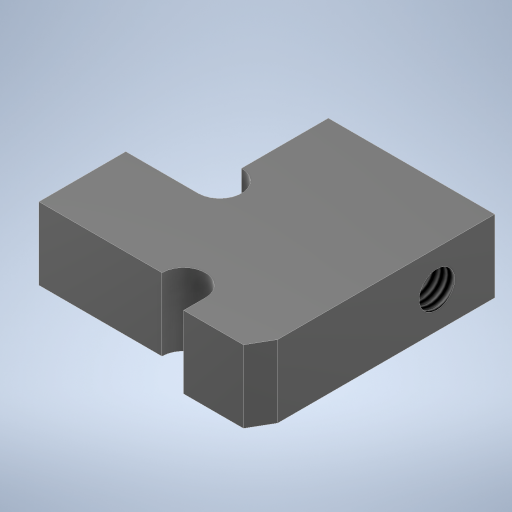
# Autodesk Inventor part: TorsoElectronicBoxLatchFrame
Saved by Autodesk Inventor 2024.2 (Build 282272000, 272)
## iProperties
Created: 2024-01-06
Part Number: TorsoElectronicBoxLatchFrame
Material: Acetal Resin, Black
Document SubType Name: Modeling
Designer: Masato Kubotera
Density: 1.425 g/cm^3
Appearance: Smooth - Black
Vendor: meviy
Mass: 1.2815 g
Surface Area: 7.94859 cm^2
Volume: 0.899295 cm^3
Author: Masato Kubotera
Autodesk Inventor part; units mm, degrees
ref_plane "YZ Plane" through (0, 0, 0) normal (1, 0, 0) x (0, 1, 0)
ref_plane "XZ Plane" through (0, 0, 0) normal (0, 1, 0) x (-1, 0, 0)
ref_plane "XY Plane" through (0, 0, 0) normal (0, 0, 1) x (1, 0, 0)
sketch "Sketch1" plane through (0, 0, 0) normal (0, 1, 0) x (-1, 0, 0)
  line L0 (0, -4) -> (0, 5)
  line L1 (0, 5) -> (5, 5)
  line L2 (5, 5) -> (5, 11)
  line L3 (5, 11) -> (-6.5, 11)
  line L4 (-6.5, 11) -> (-6.5, 12.5)
  line L5 (-6.5, 12.5) -> (-10.634, 12.5)
  line L6 (-10.634, 12.5) -> (-11.5, 11)
  line L7 (-11.5, 11) -> (-11.5, -4)
  line L8 (-11.5, -4) -> (0, -4)
  line L9 (0, 0) -> (-4.5, 0) construction
  arc A0 (0, 5) -> (0, 2) centre (0, 3.5) ccw
  arc A1 (-6.5, 11) -> (-3.5, 11) centre (-5, 11) ccw
  dimension "d0" = 5
  dimension "d1" = 6
  dimension "d2" = 15
  dimension "d3" = 4.5
  dimension "d4" = 1.5
  dimension "d5" = 1.5
  dimension "d6" = 6.5
  dimension "d7" = 30
  dimension "d8" = 5
  dimension "d18" = 4
  constraints: 20 end point, 6 point on line, 5 horizontal, 4 point on circle, 4 vertical, 2 centre point, 1 equal radius
  measures "d0" distance of L0.end L1.end
  measures "d1" distance of L1.end L2.end
  measures "d2" distance between parallel lines of L8 L3
  measures "d3" distance of L9.start L9.end
  measures "d4" radius of A0
  measures "d5" distance of L3.end L4.end
  measures "d6" distance between parallel lines of L4 L0
  measures "d7" angle of L7 L6
  measures "d8" distance between parallel lines of L4 L7
  measures "d18" distance from line of L9.start L8
extrude "Extrusion1" add sketch "Sketch1" along normal mid plane 5 contours L8 L7 L6 L5 L4 A1 L3 L2 L1 A0 L0
sketch "Sketch2" plane through (0, -2.5, 2) normal (-1, 0, 0) x (0, 0, 1)
  point P0 (-2, 2.5)
  point P1 (-2, 2.5)
  constraints: 1 coincident
hole "Hole1" at (0, 0, 0) direction (1, 0, 0) diameter 2.459 end through all thread size "M3x0.5" class "6H" standard "ANSI Metric M Profile"
body "Solid1"
